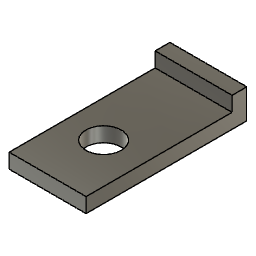
frame (Autodesk Fusion 360 design; units mm, degrees)
Autodesk Fusion 360 part; units mm, degrees
sketch "Esboço1" plane through (0, 0, 0) normal (0, 0, 1) x (1, 0, 0)
  line L0 (9, 9.5) -> (-9, 9.5)
  line L1 (-9, 9.5) -> (-9, -9.5)
  line L2 (-9, -9.5) -> (9, -9.5)
  line L3 (9, -9.5) -> (9, 9.5)
  line L4 (9, 9.5) -> (-9, -9.5) construction
  line L5 (-9, 9.5) -> (9, -9.5) construction
  line L6 (-7, -7.5) -> (7, -7.5)
  line L7 (7, -7.5) -> (7, 7.5)
  line L8 (7, 7.5) -> (-7, 7.5)
  line L9 (-7, 7.5) -> (-7, -7.5)
  dimension "d1" = 18
  dimension "d2" = 19
  dimension "d3" = -2
  constraint horizontal L0
  constraint perpendicular L0 L1
  constraint parallel L0 L2
  constraint parallel L1 L3
  constraint coincident L4 origin
  constraint coincident L5 origin
  measures "d1" distance of L1.end L2.end
  measures "d2" distance of L0.end L1.end
extrude "Extrusão1" add sketch "Esboço1" along normal blind 2 makes body 1
sketch "Esboço2" plane through (0, 0, 2) normal (0, 0, 1) x (-1, 0, 0)
  line L0 (7, 7.5) -> (7, -7.5)
  line L1 (7, -7.5) -> (-7, -7.5)
  line L2 (-7, -7.5) -> (-7, 7.5)
  line L3 (-7, 7.5) -> (7, 7.5)
  line L4 (-9, 9.5) -> (-9, -9.5)
  line L5 (-9, -9.5) -> (9, -9.5)
  line L6 (9, -9.5) -> (9, 9.5)
  line L7 (9, 9.5) -> (-9, 9.5)
  line L8 (-11, 9.5) -> (-11, -9.5)
  line L9 (-9, -11.5) -> (9, -11.5)
  line L10 (11, -9.5) -> (11, 9.5)
  line L11 (9, 11.5) -> (-9, 11.5)
  arc A0 (11, 9.5) -> (9, 11.5) centre (9, 9.5) ccw
  arc A1 (-9, 11.5) -> (-11, 9.5) centre (-9, 9.5) ccw
  arc A2 (-11, -9.5) -> (-9, -11.5) centre (-9, -9.5) ccw
  arc A3 (9, -11.5) -> (11, -9.5) centre (9, -9.5) ccw
  dimension "d7" = 2
  constraint tangent L10 A0
  constraint tangent L11 A0
  constraint tangent L11 A1
  constraint tangent L8 A1
  constraint equal A0 A1
  constraint tangent L8 A2
  constraint tangent L9 A2
  constraint equal A0 A2
  constraint tangent L10 A3
  constraint tangent L9 A3
  constraint equal A0 A3
  measures "d7" radius of A0
extrude "Extrusão2" add sketch "Esboço2" along normal blind 2 contours L4 L5 L6 L7 | L8 L9 L10 L11 A0 A1 A2 A3 bodies 1
fillet "Arredondamento1" radius 2 4 edges at (-9, 9.5, 1) (-9, -9.5, 1) (9, 9.5, 1) (9, -9.5, 1) on bodies 1
fillet "Arredondamento2" radius 1 4 edges at (-7, 7.5, 2) (-7, -7.5, 2) (7, -7.5, 2) (7, 7.5, 2) on bodies 1
sketch "Esboço3" plane through (0, 0, 0) normal (0, 0, 1) x (1, 0, 0)
  circle A0 centre (-41, 0) radius 12
  line L0 (-57.5, -16.5) -> (-24.5, -16.5)
  line L1 (-24.5, -16.5) -> (-24.5, 16.5)
  line L2 (-24.5, 16.5) -> (-57.5, 16.5)
  line L3 (-57.5, 16.5) -> (-57.5, -16.5)
  line L4 (-57.5, -16.5) -> (-24.5, 16.5) construction
  line L5 (-24.5, -16.5) -> (-57.5, 16.5) construction
  point P0 (-41, 0)
  dimension "d14" = 24
  dimension "d15" = 33
  dimension "d16" = 33
  constraint horizontal L0
  constraint perpendicular L0 L1
  constraint parallel L0 L2
  constraint parallel L1 L3
  constraint coincident L4 P0
  constraint coincident L5 P0
  constraint coincident P0 A0.centre
  measures "d14" diameter of A0
  measures "d15" distance of L1.end L2.end
  measures "d16" distance of L0.end L1.end
extrude "Extrusão3" add sketch "Esboço3" along normal blind 1 separate body makes body 2
sketch "Esboço4" plane through (0, 0, 0) normal (0, 0, 1) x (1, 0, 0)
  line L0 (73, 0) -> (53, 0)
  line L1 (53, 0) -> (53, -20)
  line L2 (53, -20) -> (73, -20)
  line L3 (73, -20) -> (73, 0)
  line L4 (63, -20) -> (63, -12)
  circle A0 centre (63, -12) radius 2.4
  dimension "d19" = 20
  dimension "d20" = 20
  dimension "d21" = 8
  dimension "d22" = 4.8
  constraint horizontal L0
  constraint vertical L1
  constraint horizontal L2
  constraint vertical L3
  constraint midpoint L2 L4.start
  constraint perpendicular L2 L4
  constraint coincident L4.end A0.centre
  measures "d19" distance of L0.start L0.end
  measures "d20" distance of L0.end L1.end
  measures "d21" distance of L4.start L4.end
  measures "d22" diameter of A0
extrude "Extrusão4" add sketch "Esboço4" along normal blind 10 separate body makes body 3
fillet "Arredondamento3" radius 6 2 edges at (73, -20, 5) (53, -20, 5) on bodies 3
sketch "Esboço5" plane through (0, 0, 10) normal (0, 0, 1) x (-1, 0, 0)
  circle A0 centre (-63, 12) radius 2.4
  arc A1 (-53, 14) -> (-59, 20) centre (-59, 14) ccw
  line L0 (-59, 20) -> (-67, 20)
  arc A2 (-67, 20) -> (-73, 14) centre (-67, 14) ccw
  line L1 (-73, 14) -> (-73, 0)
  line L2 (-73, 0) -> (-53, 0)
  line L3 (-53, 0) -> (-53, 14)
  line L4 (-53, 0) -> (-73, 0)
  line L5 (-73, 0) -> (-73, -2)
  line L6 (-73, -2) -> (-53, -2)
  line L7 (-53, -2) -> (-53, 0)
  dimension "d27" = 2
  constraint horizontal L4
  constraint vertical L5
  constraint horizontal L6
  constraint vertical L7
  constraint coincident L2.end L3.start
  measures "d27" distance of L2.end L6.end
extrude "Extrusão5" add sketch "Esboço5" along normal blind 2 from surface at 1 separate body makes body 4
sketch "Esboço6" plane through (0, 0, 13) normal (0, 0, 1) x (-1, 0, 0)
  circle A0 centre (-63, 12) radius 2.4
  line L0 (-53, -2) -> (-53, 14)
  arc A1 (-53, 14) -> (-59, 20) centre (-59, 14) ccw
  line L1 (-59, 20) -> (-67, 20)
  arc A2 (-67, 20) -> (-73, 14) centre (-67, 14) ccw
  line L2 (-73, 14) -> (-73, -2)
  line L3 (-73, -2) -> (-53, -2)
  line L4 (-53, -2) -> (-73, -2)
  line L5 (-73, -2) -> (-73, 0)
  line L6 (-73, 0) -> (-53, 0)
  line L7 (-53, 0) -> (-53, -2)
  constraint horizontal L4
  constraint vertical L5
  constraint horizontal L6
  constraint vertical L7
  constraint coincident L2 L5.end
  constraint coincident L0.start L3.end
extrude "Extrusão6" add sketch "Esboço6" along normal blind 2 contours L0 L2 L3 L4 L5 L6 L7 bodies 4
sketch "Esboço7" plane through (0, 0, 11) normal (0, 0, -1) x (1, 0, 0)
  circle A0 centre (63, 12) radius 2.4
  line L0 (53, 14) -> (53, -2)
  line L1 (53, -2) -> (73, -2)
  line L2 (73, -2) -> (73, 14)
  arc A1 (73, 14) -> (67, 20) centre (67, 14) ccw
  line L3 (67, 20) -> (59, 20)
  arc A2 (59, 20) -> (53, 14) centre (59, 14) ccw
  line L4 (58, -2) -> (68.4479, -2)
  line L5 (68.4479, -2) -> (68.4479, 19.8227)
  line L6 (68.4479, 19.8227) -> (58, 19.8227)
  line L7 (58, 19.8227) -> (58, -2)
  constraint horizontal L4
  constraint vertical L5
  constraint horizontal L6
  constraint vertical L7
  constraint coincident A1 L5.end
  constraint coincident L1 L4.start
extrude "Extrusão7" cut sketch "Esboço7" against normal blind 10 contours L0 L1 A1 L3 A2 L6 L7 | L1 L2 A1 L5 bodies 4
hidden bodies 1 2 3
